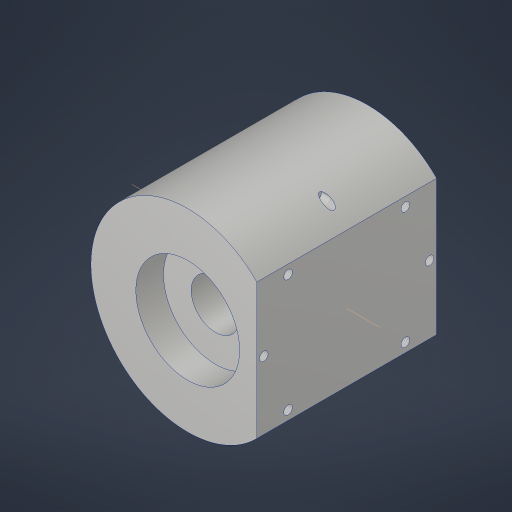
# Autodesk Inventor part: EL2-A-004
Saved by Autodesk Inventor 2023.4 (Build 274418000, 418)
## iProperties
Created: 2025-01-12
Part Number: EL2-A-004
Material: Aluminum 6061
Document SubType Name: Modeling
Designer: brand
Density: 2.7 g/cm^3
Appearance: Aluminum - Flat
Author: brand
Autodesk Inventor part; units mm, degrees
ref_plane "YZ Plane" through (0, 0, 0) normal (1, 0, 0) x (0, 1, 0)
ref_plane "XZ Plane" through (0, 0, 0) normal (0, 1, 0) x (-1, 0, 0)
ref_plane "XY Plane" through (0, 0, 0) normal (0, 0, 1) x (1, 0, 0)
sketch "Sketch1" plane through (0, 0, 0) normal (0, 0, 1) x (1, 0, 0)
  circle A0 centre (0, 0) radius 11.1125
  circle A1 centre (0, 0) radius 57.15 construction
  line L0 (29.571, 44.45) -> (35.921, 44.45) construction
  line L1 (35.921, 44.45) -> (35.921, -44.45) construction
  line L2 (35.921, -44.45) -> (29.571, -44.45) construction
  line L3 (29.571, -44.45) -> (29.571, 44.45) construction
  line L4 (31.75, 47.519) -> (31.75, -47.519)
  arc A2 (31.75, 47.519) -> (31.75, -47.519) centre (0, 0) ccw
  point P0 (29.571, 0)
  point P1 (57.15, 0)
  point P2 (35.921, 0)
  dimension "d0" = 22.225
  dimension "d2" = 114.3
  dimension "d3" = 88.9
  dimension "d4" = 6.35
  dimension "d5" = 35.921
  dimension "d6" = 21.229
  dimension "d7" = 31.75
  constraints: 10 end point, 4 point on circle, 3 centre point, 3 coincident, 2 horizontal alignment, 2 midpoint, 2 parallel, 1 concentric, 1 horizontal, 1 perpendicular, 1 vertical
  measures "d0" diameter of A0
  measures "d2" diameter of A1
  measures "d3" distance of L2.end L0.start
  measures "d4" distance of L0.start L0.end
  measures "d5" distance from line of point (0, 0) L1
  measures "d6" distance of A1.end point (35.921, 0)
  measures "d7" distance from line of L4 point (0, 0)
extrude "Extrusion1" add sketch "Sketch1" along normal mid plane 82.55
sketch "Sketch3" plane through (0, 0, 41.275) normal (0, 0, 1) x (1, 0, 0)
  circle A0 centre (0, 0) radius 11.1125 construction
  arc A1 (31.75, 47.519) -> (31.75, -47.519) centre (0, 0) ccw construction
  line L0 (31.75, 47.519) -> (31.75, -47.519) construction
  circle A2 centre (0, 0) radius 11.1125 construction
  circle A3 centre (0, 0) radius 23.8125
  dimension "d10" = 47.625
  constraints: 1 centre point, 1 coincident
  measures "d10" diameter of A3
extrude "Extrusion2" cut sketch "Sketch3" against normal blind 12.7
sketch "Sketch4" plane through (0, 0, -41.275) normal (0, 0, -1) x (-1, 0, 0)
  circle A0 centre (0, 0) radius 23.8125
  dimension "d13" = 47.625
  constraints: 1 centre point, 1 coincident
  measures "d13" diameter of A0
extrude "Extrusion3" cut sketch "Sketch4" against normal blind 12.7
sketch "Sketch5" plane through (31.75, -47.519, 41.275) normal (1, 0, 0) x (0, 0, -1)
  line L0 (82.55, 95.0381) -> (82.55, 0) construction
  line L1 (82.55, 0) -> (0, 0) construction
  line L2 (0, 0) -> (0, 95.0381) construction
  line L3 (0, 95.0381) -> (82.55, 95.0381) construction
  circle A0 centre (41.275, 47.519) radius 38.1 construction
  point P0 (41.275, 85.619)
  dimension "d16" = 76.2
  constraints: 2 vertical alignment, 1 coincident, 2 other
hole "Hole1" at (31.75, 38.1, 0) direction (-1, 0, 0) diameter 3.9624 depth 13.6144 thread size "10-32 UNF" class "2B" standard "ANSI Unified Screw Threads"
pattern_circular "Circular Pattern1" count 8 over 360 about axis through (31.75, 0, 0) along (1, 0, 0) of "Hole1"
sketch "Sketch6" plane through (0, 0, 41.275) normal (0, 0, 1) x (1, 0, 0)
  circle A0 centre (0, 0) radius 23.8125 construction
  arc A1 (31.75, 47.519) -> (31.75, -47.519) centre (0, 0) ccw construction
  line L0 (31.75, 47.519) -> (31.75, -47.519) construction
  circle A2 centre (0, 0) radius 44.45
  circle A3 centre (0, 0) radius 57.15
  arc A4 (31.75, 47.519) -> (31.75, -47.519) centre (0, 0) ccw construction
  dimension "d27" = 12.7
  constraints: 2 centre point, 2 coincident, 1 concentric
  measures "d27" radial gap between concentric circles of A1 A2
extrude "Extrusion4" cut sketch "Sketch6" against normal through all
equation "\"d13\" = d10"
equation "\"d14\" = d11"
equation "\"d11\" = 12.7"
body "Solid1"
